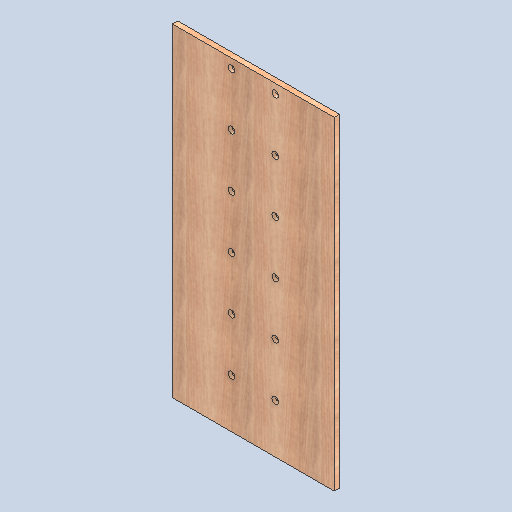
# Autodesk Inventor part: IMS-00-003
Saved by Autodesk Inventor 2022 (Build 260153000, 153)
## iProperties
Created: 2020-10-22
Part Number: IMS-00-003
Material: Wood (Birch)
Document SubType Name: Sheet Metal
Designer: mahra
Mass: 8167.09 g
Surface Area: 15664.8 cm^2
Volume: 14849.2 cm^3
Density: 0.55 g/cm^3
Appearance: Birch - Natural Polished
Sheet Metal Rule: Default
Author: mahra
Autodesk Inventor part; units mm, degrees
ref_plane "YZ Plane" through (0, 0, 0) normal (1, 0, 0) x (0, 1, 0)
ref_plane "XZ Plane" through (0, 0, 0) normal (0, 1, 0) x (-1, 0, 0)
ref_plane "XY Plane" through (0, 0, 0) normal (0, 0, 1) x (1, 0, 0)
sketch "Sketch1" plane through (0, 0, 0) normal (0, 0, 1) x (1, 0, 0)
  line L0 (-305, 610) -> (305, 610)
  line L1 (305, 610) -> (305, -610)
  line L2 (305, -610) -> (-305, -610)
  line L3 (-305, -610) -> (-305, 610)
  line L4 (-305, 610) -> (305, -610) construction
  line L5 (305, 610) -> (-305, -610) construction
  point P0 (0, 0)
  dimension "d0" = 610
  dimension "d1" = 1220
  constraints: 12 end point, 2 midpoint, 2 parallel, 1 horizontal, 1 perpendicular
  measures "d0" distance of L1.end L2.end
  measures "d1" distance of L2.end L0.start
extrude "Extrusion1" add sketch "Sketch1" along normal blind 20
sketch "Sketch2" plane through (0, 0, 20) normal (0, 0, 1) x (1, 0, 0)
  circle A0 centre (82.5, 575) radius 5 projected
  circle A1 centre (82.5, -25) radius 5 projected
  circle A2 centre (82.5, 375) radius 5 projected
  circle A3 centre (82.5, -225) radius 5 projected
  circle A4 centre (82.5, 175) radius 5 projected
  arc A5 (92.5, -250) -> (97.5, -245) centre (92.5, -245) ccw projected
  line L0 (69.5, -250) -> (92.5, -250) projected
  line L1 (69.5, -250) -> (69.5, 600) projected
  line L2 (92.5, 600) -> (69.5, 600) projected
  arc A6 (97.5, 595) -> (92.5, 600) centre (92.5, 595) ccw projected
  line L3 (97.5, -245) -> (97.5, 595) projected
  circle A7 centre (-82.5, 575) radius 5 projected
  circle A8 centre (-82.5, -25) radius 5 projected
  circle A9 centre (-82.5, 375) radius 5 projected
  circle A10 centre (-82.5, -225) radius 5 projected
  circle A11 centre (-82.5, 175) radius 5 projected
  arc A12 (-97.5, -245) -> (-92.5, -250) centre (-92.5, -245) ccw projected
  line L4 (-97.5, 595) -> (-97.5, -245) projected
  arc A13 (-92.5, 600) -> (-97.5, 595) centre (-92.5, 595) ccw projected
  line L5 (-69.5, 600) -> (-92.5, 600) projected
  line L6 (-69.5, -250) -> (-69.5, 600) projected
  line L7 (-92.5, -250) -> (-69.5, -250) projected
  point P0 (0, 0)
extrude "Extrusion2" cut sketch "Sketch2" against normal through all contours A0 | A1 | A2 | A3 | A4 | A7 | A8 | A9 | A10 | A11
sketch "Sketch3" plane through (0, 0, 20) normal (0, 0, 1) x (1, 0, 0)
  circle A0 centre (-82.5, 575) radius 5 projected
  point P0 (0, 0)
  constraints: 1 coincident
hole "Hole1" at (-82.5, 575, 20) direction (0, 0, -1) diameter 8 end through all countersink diameter 25 countersink angle 90
mirror "Mirror1" about plane through (0, 0, 0) normal (1, 0, 0) of "Hole1"
pattern_linear "Rectangular Pattern1" count 6 spacing 200 along (0, -1, 0) of "Hole1", "Mirror1"
sketch "Sketch4" plane through (0, 0, 20) normal (0, 0, 1) x (1, 0, 0)
  circle A0 centre (82.5, -425) radius 5 projected
  circle A1 centre (-82.5, -425) radius 5 projected
  point P0 (0, 0)
extrude "Extrusion3" cut sketch "Sketch4" against normal through all
equation "\"BendRadius\" = Thickness"
equation "\"BendReliefWidth\" = Thickness"
equation "\"BendReliefDepth\" = 0.5 * Thickness"
equation "\"CornerReliefSize\" = 4 * Thickness"
equation "\"MinimumRemnant\" = 2 * Thickness"
equation "\"TransitionRadius\" = BendRadius"
equation "\"JacobiRadiusSize\" = Thickness"
equation "\"GapSize\" = Thickness"
equation "\"Thickness\" = 0.5"
body "Solid1"
